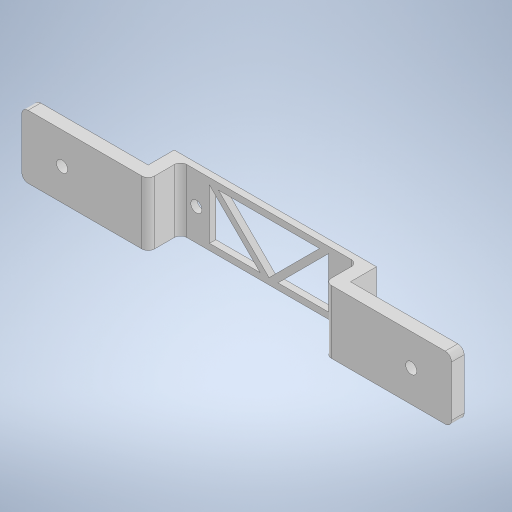
# Autodesk Inventor part: axis3
Saved by Autodesk Inventor 2023 (Build 270158000, 158)
## iProperties
Created: 2023-04-29
Part Number: axis3
Material: 一般
Document SubType Name: Modeling
Designer: taka2
Density: 1 g/cm^3
Appearance: 既定
Author: taka2
Autodesk Inventor part; units mm, degrees
ref_plane "YZ Plane" through (0, 0, 0) normal (1, 0, 0) x (0, 1, 0)
ref_plane "XZ Plane" through (0, 0, 0) normal (0, 1, 0) x (-1, 0, 0)
ref_plane "XY Plane" through (0, 0, 0) normal (0, 0, 1) x (1, 0, 0)
sketch "スケッチ1" plane through (0, 0, 0) normal (0, 1, 0) x (-1, 0, 0)
  line L0 (0, 20.7547) -> (0, -42.4528)
  line L1 (68, 12.25) -> (28, 12.25)
  line L2 (28, 12.25) -> (28, 2)
  line L3 (28, 2) -> (0, 2)
  line L4 (68, 12.25) -> (68, 8.25)
  line L5 (68, 8.25) -> (32, 8.25)
  line L6 (32, 8.25) -> (32, 0)
  line L7 (32, 0) -> (0, 0)
  line L8 (-68, 12.25) -> (-28, 12.25)
  line L9 (-28, 12.25) -> (-28, 2)
  line L10 (-28, 2) -> (0, 2)
  line L11 (-68, 12.25) -> (-68, 8.25)
  line L12 (-68, 8.25) -> (-32, 8.25)
  line L13 (-32, 8.25) -> (-32, 0)
  line L14 (-32, 0) -> (0, 0)
  dimension "d0" = 40
  dimension "d1" = 4
  dimension "d2" = 36
  dimension "d3" = 10.25
  dimension "d4" = 2
  dimension "d5" = 56
  constraints: 30 end point, 6 symmetric about line, 5 perpendicular, 4 point on line, 2 vertical, 1 horizontal
  measures "d0" distance of L1.start L1.end
  measures "d1" distance of L1.start L4.end
  measures "d2" distance of L4.end L5.end
  measures "d3" distance of L1.end L2.end
  measures "d4" distance between parallel lines of L3 L7
  measures "d5" distance of L9.end L2.end
extrude "押し出し1" add sketch "スケッチ1" along normal blind 20
sketch "スケッチ2" plane through (32, 0, 0) normal (0, 0, -1) x (-1, 0, 0)
  line L0 (0, 0) -> (0, 20) projected
  line L1 (0, 10) -> (64, 10)
  line L2 (64, 0) -> (64, 20) projected
  line L3 (32, 0) -> (32, 20)
  line L4 (0, 20) -> (64, 20) projected
  circle A0 centre (9, 10) radius 1.75
  line L5 (13.1716, 18) -> (13.1716, 2)
  line L6 (13.1716, 2) -> (29.1716, 2)
  line L7 (29.1716, 2) -> (13.1716, 18)
  line L8 (16, 18) -> (32, 18)
  line L9 (16, 18) -> (32, 2)
  circle A1 centre (55, 10) radius 1.75
  line L10 (50.8284, 18) -> (50.8284, 2)
  line L11 (50.8284, 2) -> (34.8284, 2)
  line L12 (34.8284, 2) -> (50.8284, 18)
  line L13 (48, 18) -> (32, 18)
  line L14 (48, 18) -> (32, 2)
  dimension "d8" = 16
  dimension "d9" = 3.5
  dimension "d10" = 2
  dimension "d11" = 46
  constraints: 24 end point, 7 symmetric about line, 3 midpoint, 3 point on line, 2 centre point, 2 equal length, 2 vertical, 1 horizontal, 1 parallel, 1 perpendicular, 1 other
  measures "d8" distance of L5.start L5.end
  measures "d9" diameter of A0
  measures "d10" distance between parallel lines of L7 L9
  measures "d11" distance of A1.centre A0.centre
extrude "押し出し2" cut sketch "スケッチ2" against normal through all contours A0 L1 | L1 A0 | L13 L14 L1 L3 | L3 L1 L9 L8 | L5 L7 L1 | L1 L7 L6 L5 | L3 L9 L1 | L1 L14 L3 | A1 L1 | L1 A1 | L12 L10 L1 | L1 L10 L11 L12
sketch "スケッチ3" plane through (28, 0, 12.25) normal (0, 0, 1) x (1, 0, 0)
  line L0 (-96, 0) -> (-96, 20) projected
  line L1 (-96, 10) -> (40, 10)
  line L2 (40, 0) -> (40, 20) projected
  circle A0 centre (27.25, 10) radius 1.75
  circle A1 centre (-83.25, 10) radius 1.75
  point P0 (-28, 0)
  dimension "d14" = 3.5
  dimension "d15" = 12.75
  dimension "d16" = 12.75
  constraints: 2 centre point, 2 end point, 2 midpoint, 2 point on line, 1 equal radius
  measures "d14" diameter of A0
  measures "d15" distance from line of L2 A0.centre
  measures "d16" distance from line of L0 A1.centre
extrude "押し出し3" cut sketch "スケッチ3" against normal through all
fillet "フィレット1" radius 2 4 edges at (-68, 20, 10.25) (68, 20, 10.25) (68, 0, 10.25) (-68, 0, 10.25)
fillet "フィレット2" radius 2 4 edges at (-28, 10, 2) (-28, 10, 12.25) (28, 10, 2) (28, 10, 12.25)
